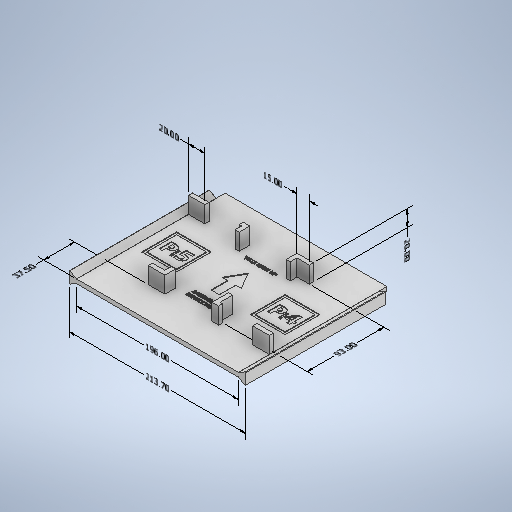
# Autodesk Inventor part: Suelo2
Saved by Autodesk Inventor 2025.1 (Build 291241000, 241)
## iProperties
Created: 2025-11-20
Part Number: Suelo2
Material: Genérico
Document SubType Name: Modeling
Designer: Diego
Density: 1 g/cm^3
Appearance: Valor por defecto
Author: Diego
Autodesk Inventor part; units mm, degrees
(part 1 of 2)
ref_plane "YZ Plane" through (0, 0, 0) normal (1, 0, 0) x (0, 1, 0)
ref_plane "XZ Plane" through (0, 0, 0) normal (0, 1, 0) x (-1, 0, 0)
ref_plane "XY Plane" through (0, 0, 0) normal (0, 0, 1) x (1, 0, 0)
sketch "Boceto1" plane through (0, 0, 0) normal (0, 0, 1) x (1, 0, 0)
  line L0 (-107.4375, 9.96) -> (-116.4375, 15.1562)
  line L1 (-116.4375, 15.1562) -> (-116.4375, -0.2361)
  line L2 (-116.4375, -0.2361) -> (-107.4375, 4.96)
  line L3 (-107.4375, 9.96) -> (-98.4042, 9.96) construction
  line L4 (-107.4375, 4.96) -> (-97.9616, 4.96) construction
  line L5 (-107.4375, 12.46) -> (-107.4375, 9.96) construction
  line L6 (-107.4375, 12.46) -> (-107.4375, 9.96) construction
  line L7 (-107.4375, 2.46) -> (-107.4375, 4.96) construction
  line L8 (88.5625, 12.46) -> (88.5625, 9.96) construction
  line L9 (88.5625, 12.46) -> (88.5625, 9.96) construction
  line L10 (97.5625, -0.2361) -> (88.5625, 4.96)
  line L11 (88.5625, 9.96) -> (97.5625, 15.1562)
  line L12 (97.5625, 15.1562) -> (97.5625, -0.2361)
  line L13 (88.5625, 4.96) -> (88.5625, 4.96) construction
  line L14 (88.5625, 4.96) -> (88.5625, 4.96) construction
  line L15 (88.5625, 4.96) -> (88.5625, 4.96)
  line L16 (88.5625, 7.46) -> (88.5625, 4.96)
  line L17 (88.5625, 4.96) -> (88.5625, 4.96)
  line L18 (88.5625, 9.96) -> (88.5625, 7.46)
  line L19 (-107.4375, 9.96) -> (-107.4375, 4.96)
  point P0 (0, 0)
  point P1 (-116.4375, 7.46)
  point P2 (97.5625, 7.46)
  point P3 (93.0625, 12.5581)
  point P4 (-111.9375, 12.5581)
  dimension "d0" = 60
  constraints: 40 end point, 5 vertical, 3 midpoint, 2 horizontal, 1 collinear, 1 parallel, 5 other
  measures "d0" angle of L0 L1
extrude "Extrusión1" add sketch "Boceto1" against normal blind 170
sketch "Boceto2" plane through (0, 0, 0) normal (0, 0, 1) x (1, 0, 0)
  line L0 (-107.4375, 9.96) -> (-107.4375, 4.96) projected
  line L1 (97.5625, -0.2361) -> (88.5625, 4.96) projected
  line L2 (-107.4375, 9.96) -> (88.5625, 9.96)
  line L3 (88.5625, 9.96) -> (88.5625, 4.96)
  line L4 (88.5625, 4.96) -> (-107.4375, 4.96)
  line L5 (-107.4375, 4.96) -> (-107.4375, 9.96)
  point P0 (0, 0)
  constraints: 8 end point, 2 parallel, 1 horizontal, 1 perpendicular
extrude "Extrusión2" add sketch "Boceto2" against normal blind 180
sketch "Boceto3" plane through (-107.4375, 9.96, 0) normal (0, 1, 0) x (1, 0, 0)
  line L0 (0, 0) -> (196, 0) projected
  line L1 (0, 0) -> (0, 170) projected
  line L2 (0, 180) -> (64.5, 180) construction
  line L3 (64.5, 42.5) -> (0, 42.5) construction
  line L4 (0, 42.5) -> (0, 180) construction
  line L5 (0, 180) -> (196, 180) projected
  line L6 (0, 170) -> (0, 180) projected
  line L7 (196, 180) -> (0, 180) construction
  line L8 (98, 180) -> (98, 0) construction
  line L9 (64.5, 89) -> (0, 89) construction
  line L10 (32.25, 180) -> (32.25, 42.5) construction
  line L11 (64.5, 107) -> (0, 107) construction
  line L12 (64.5, 71) -> (0, 71) construction
  line L13 (64.5, 42.5) -> (64.5, 50.5)
  line L14 (64.5, 50.5) -> (69.5, 50.5)
  line L15 (69.5, 50.5) -> (69.5, 37.5)
  line L16 (69.5, 37.5) -> (49.5, 37.5)
  line L17 (49.5, 37.5) -> (49.5, 42.5)
  line L18 (49.5, 42.5) -> (64.5, 42.5)
  line L19 (64.5, 135.5) -> (64.5, 127.5)
  line L20 (64.5, 127.5) -> (69.5, 127.5)
  line L21 (69.5, 127.5) -> (69.5, 140.5)
  line L22 (69.5, 140.5) -> (64.5, 140.5)
  line L23 (131.5, 42.5) -> (131.5, 57.5)
  line L24 (131.5, 57.5) -> (126.5, 57.5)
  line L25 (126.5, 57.5) -> (126.5, 37.5)
  line L26 (126.5, 37.5) -> (134.5, 37.5)
  line L27 (134.5, 37.5) -> (134.5, 42.5)
  line L28 (134.5, 42.5) -> (131.5, 42.5)
  line L29 (131.5, 127.5) -> (126.5, 127.5)
  line L30 (131.5, 135.5) -> (131.5, 127.5)
  line L31 (146.5, 135.5) -> (131.5, 135.5)
  line L32 (126.5, 135.5) -> (126.5, 140.5)
  line L33 (146.5, 140.5) -> (146.5, 135.5)
  line L34 (126.5, 140.5) -> (146.5, 140.5)
  line L35 (146.5, 140.5) -> (-13.2396, 140.5) construction
  line L36 (0, 140.5) -> (20, 140.5)
  line L37 (20, 140.5) -> (20, 135.5)
  line L38 (20, 135.5) -> (0, 135.5)
  line L39 (0, 135.5) -> (0, 140.5)
  line L40 (64.5, 140.5) -> (61.5, 140.5)
  line L41 (61.5, 140.5) -> (61.5, 135.5)
  line L42 (61.5, 135.5) -> (64.5, 135.5)
  line L43 (64.5, 180) -> (64.5, 140.5) construction
  line L44 (64.5, 135.5) -> (64.5, 42.5) construction
  line L45 (126.5, 135.5) -> (126.5, 127.5)
  line L46 (196, 140.5) -> (176, 140.5) construction
  line L47 (176, 140.5) -> (176, 135.5) construction
  line L48 (176, 135.5) -> (196, 135.5) construction
  line L49 (176, 37.5) -> (176, 42.5)
  line L50 (176, 42.5) -> (196, 42.5)
  line L51 (196, 37.5) -> (176, 37.5)
  line L52 (196, 37.5) -> (196, 42.5)
  point P0 (107.4375, 0)
  point P1 (0, 135.5)
  dimension "d14" = 36
  dimension "d21" = 37.5
  dimension "d22" = 5
  dimension "d23" = 20
  dimension "d24" = 5
  dimension "d25" = 64.5
  dimension "d26" = 13
  dimension "d27" = 46.5
  dimension "d54" = 39.5
  dimension "d60" = 93
  dimension "d76" = 20
  dimension "d77" = 5
  dimension "d81" = 3
  dimension "d82" = 5
  dimension "d83" = 20
  dimension "d84" = 15
  dimension "d85" = 5
  dimension "d89" = 5
  dimension "d90" = 5
  dimension "d93" = 15
  dimension "d94" = 8
  dimension "d95" = 3
  dimension "d97" = 28.5
  dimension "d98" = 5
  dimension "d99" = 5
  constraints: 96 end point, 16 perpendicular, 13 point on line, 11 symmetric about line, 8 horizontal, 6 parallel, 5 midpoint, 5 vertical, 3 collinear, 1 other
  measures "d14" distance between parallel lines of L12 L11
  measures "d21" distance between parallel lines of L0 L16
  measures "d22" distance of L16.end L17.end
  measures "d23" distance of L15.end L16.end
  measures "d24" distance of L13.end L14.end
  measures "d25" distance between parallel lines of L1 L13
  measures "d26" distance of L14.end L15.end
  measures "d27" distance between parallel lines of L18 L9
  measures "d54" distance between parallel lines of L5 L22
  measures "d60" distance between parallel lines of L28 L31
  measures "d76" distance of L37.end L38.end
  measures "d77" distance of L36.end L37.end
  measures "d81" distance of L19.start L41.end
  measures "d82" distance of L40.end L41.end
  measures "d83" distance of L24.end L26.start
  measures "d84" distance of L23.start L24.start
  measures "d85" distance of L24.start L24.end
  measures "d89" distance of L32.start L32.end
  measures "d90" distance of L34.end L31.start
  measures "d93" distance of L31.start L30.start
  measures "d94" distance of L30.start L30.end
  measures "d95" distance of L28.start L23.start
  measures "d97" distance between parallel lines of L8 L25
  measures "d98" distance of L29.start L29.end
  measures "d99" distance of L27.start L28.start
sketch "Boceto4" plane through (-107.4375, 9.96, 0) normal (0, 1, 0) x (1, 0, 0)
  line L0 (12.9564, 122.5347) -> (51.5436, 122.5347) construction
  line L1 (51.5436, 122.5347) -> (51.5436, 55.4653) construction
  line L2 (51.5436, 55.4653) -> (12.9564, 55.4653) construction
  line L3 (12.9564, 55.4653) -> (12.9564, 122.5347) construction
  line L4 (64.5, 107) -> (0, 107) construction
  line L5 (64.5, 89) -> (0, 89) construction
  line L6 (64.5, 71) -> (0, 71) construction
  line L7 (64.5, 180) -> (64.5, 42.5) construction
  line L8 (32.25, 180) -> (32.25, 42.5) construction
  line L9 (98, 180) -> (98, 0) construction
  line L10 (131.5, 107) -> (196, 107) construction
  line L11 (131.5, 89) -> (196, 89) construction
  line L12 (131.5, 71) -> (196, 71) construction
  line L13 (163.75, 180) -> (163.75, 42.5) construction
  line L14 (149.758, 125.112) -> (177.742, 125.112) construction
  line L15 (177.742, 125.112) -> (177.742, 52.888) construction
  line L16 (177.742, 52.888) -> (149.758, 52.888) construction
  line L17 (149.758, 52.888) -> (149.758, 125.112) construction
  line L18 (131.5, 180) -> (131.5, 42.5) construction
  line L19 (14.25, 71) -> (50.25, 71)
  line L20 (50.25, 71) -> (50.25, 107)
  line L21 (50.25, 107) -> (14.25, 107)
  line L22 (14.25, 107) -> (14.25, 71)
  line L23 (14.25, 71) -> (50.25, 107) construction
  line L24 (50.25, 71) -> (14.25, 107) construction
  line L25 (11.25, 68) -> (53.25, 68)
  line L26 (53.25, 68) -> (53.25, 110)
  line L27 (53.25, 110) -> (11.25, 110)
  line L28 (11.25, 110) -> (11.25, 68)
  line L29 (181.75, 71) -> (145.75, 71)
  line L30 (145.75, 71) -> (145.75, 107)
  line L31 (145.75, 107) -> (181.75, 107)
  line L32 (181.75, 107) -> (181.75, 71)
  line L33 (181.75, 71) -> (145.75, 107) construction
  line L34 (145.75, 71) -> (181.75, 107) construction
  line L35 (184.75, 68) -> (142.75, 68)
  line L36 (142.75, 68) -> (142.75, 110)
  line L37 (142.75, 110) -> (184.75, 110)
  line L38 (184.75, 110) -> (184.75, 68)
  line L39 (93, 90) -> (93, 70)
  line L40 (93, 70) -> (103, 70)
  line L41 (103, 70) -> (103, 90)
  line L42 (103, 90) -> (93, 70) construction
  line L43 (93, 90) -> (103, 70) construction
  line L44 (93, 90) -> (86.453, 90)
  line L45 (86.453, 90) -> (98, 110)
  line L46 (98, 110) -> (109.547, 90)
  line L47 (109.547, 90) -> (103, 90)
  line L48 (196, 0) -> (0, 0) projected
  line L49 (74.4962, 55) -> (125.486, 55) construction
  line L50 (82.3818, 77.2089) -> (113.6182, 77.2089) construction
  line L51 (113.6182, 77.2089) -> (113.6182, 32.7911) construction
  line L52 (113.6182, 32.7911) -> (82.3818, 32.7911) construction
  line L53 (82.3818, 32.7911) -> (82.3818, 77.2089) construction
  line L54 (76.287, 55) -> (119.713, 55) construction
  line L55 (98, 110) -> (98, 70) construction
  line L56 (76.287, 125) -> (119.713, 125) construction
  line L57 (78.0417, 136.6375) -> (117.9583, 136.6375) construction
  line L58 (117.9583, 136.6375) -> (117.9583, 113.3625) construction
  line L59 (117.9583, 113.3625) -> (78.0417, 113.3625) construction
  line L60 (78.0417, 113.3625) -> (78.0417, 136.6375) construction
  spline S0 degree 2 poles (29.9202, 91.9295) (29.9202, 90.8841) (29.2516, 88.9878) (28.6317, 88.3558) knots 0 0 0 1 2 2 2
  spline S1 degree 2 poles (28.6317, 88.3558) (28.2549, 87.9546) (27.331, 87.2982) (26.784, 87.0673) knots 0 0 0 1 2 2 2
  spline S2 degree 2 poles (26.784, 87.0673) (26.2249, 86.8363) (24.9242, 86.5689) (24.122, 86.5689) knots 0 0 0 1 2 2 2
  line L61 (24.122, 86.5689) -> (22.1528, 86.5689)
  line L62 (22.1528, 86.5689) -> (22.1528, 81.658)
  line L63 (22.1528, 81.658) -> (18.3845, 81.658)
  line L64 (18.3845, 81.658) -> (18.3845, 96.658)
  line L65 (18.3845, 96.658) -> (24.2071, 96.658)
  spline S3 degree 2 poles (24.2071, 96.658) (25.4955, 96.658) (27.3797, 96.184) (28.1455, 95.6734) knots 0 0 0 1 2 2 2
  spline S4 degree 2 poles (28.1455, 95.6734) (28.9964, 95.1021) (29.9202, 93.2301) (29.9202, 91.9295) knots 0 0 0 1 2 2 2
  spline S5 degree 2 poles (26.0547, 91.8323) (26.0547, 92.4765) (25.4469, 93.3882) (25.0336, 93.5583) knots 0 0 0 1 2 2 2
  spline S6 degree 2 poles (25.0336, 93.5583) (24.4988, 93.7893) (23.5263, 93.8622) (22.6876, 93.8622) knots 0 0 0 1 2 2 2
  line L66 (22.6876, 93.8622) -> (22.1528, 93.8622)
  line L67 (22.1528, 93.8622) -> (22.1528, 89.3647)
  line L68 (22.1528, 89.3647) -> (22.4202, 89.3647)
  spline S7 degree 2 poles (22.4202, 89.3647) (22.9429, 89.3647) (23.891, 89.389) (24.2435, 89.4498) knots 0 0 0 1 2 2 2
  spline S8 degree 2 poles (24.2435, 89.4498) (24.5474, 89.4984) (25.216, 89.7901) (25.3983, 89.9724) knots 0 0 0 1 2 2 2
  spline S9 degree 2 poles (25.3983, 89.9724) (25.7873, 90.3371) (26.0547, 91.1515) (26.0547, 91.8323) knots 0 0 0 1 2 2 2
  line L69 (33.6317, 81.658) -> (31.2816, 81.658)
  line L70 (31.2816, 81.658) -> (31.2816, 89.2026)
  line L71 (31.2816, 89.2026) -> (33.6317, 89.2026)
  line L72 (33.6317, 89.2026) -> (33.6317, 81.658)
  line L73 (33.7046, 90.2804) -> (31.2168, 90.2804)
  line L74 (31.2168, 90.2804) -> (31.2168, 92.1118)
  line L75 (31.2168, 92.1118) -> (33.7046, 92.1118)
  line L76 (33.7046, 92.1118) -> (33.7046, 90.2804)
  spline S10 degree 2 poles (46.7354, 86.7391) (46.7354, 85.56) (45.9331, 83.5665) (45.143, 82.8493) knots 0 0 0 1 2 2 2
  spline S11 degree 2 poles (45.143, 82.8493) (44.3529, 82.1321) (42.1892, 81.342) (40.609, 81.342) knots 0 0 0 1 2 2 2
  spline S12 degree 2 poles (40.609, 81.342) (38.9315, 81.3541) (36.5247, 81.9011) (35.7346, 82.2536) knots 0 0 0 1 2 2 2
  line L77 (35.7346, 82.2536) -> (35.7346, 85.5235)
  line L78 (35.7346, 85.5235) -> (36.075, 85.5235)
  spline S13 degree 2 poles (36.075, 85.5235) (36.3667, 85.3655) (37.0717, 84.9522) (37.643, 84.7334) knots 0 0 0 1 2 2 2
  spline S14 degree 2 poles (37.643, 84.7334) (38.1779, 84.5267) (39.284, 84.2472) (39.9526, 84.2472) knots 0 0 0 1 2 2 2
  spline S15 degree 2 poles (39.9526, 84.2472) (40.5361, 84.2472) (41.8975, 84.5389) (42.3108, 84.9279) knots 0 0 0 1 2 2 2
  spline S16 degree 2 poles (42.3108, 84.9279) (42.6147, 85.2318) (42.955, 85.9733) (42.955, 86.5932) knots 0 0 0 1 2 2 2
  spline S17 degree 2 poles (42.955, 86.5932) (42.955, 87.128) (42.5174, 87.8817) (42.1649, 88.1126) knots 0 0 0 1 2 2 2
  spline S18 degree 2 poles (42.1649, 88.1126) (41.6544, 88.453) (40.1957, 88.6475) (39.673, 88.6475) knots 0 0 0 1 2 2 2
  spline S19 degree 2 poles (39.673, 88.6475) (38.8464, 88.6475) (37.2784, 88.3801) (36.7071, 88.2342) knots 0 0 0 1 2 2 2
  line L79 (36.7071, 88.2342) -> (36.3788, 88.2342)
  line L80 (36.3788, 88.2342) -> (36.3788, 96.658)
  line L81 (36.3788, 96.658) -> (46.3221, 96.658)
  line L82 (46.3221, 96.658) -> (46.3221, 93.8258)
  line L83 (46.3221, 93.8258) -> (39.9404, 93.8258)
  line L84 (39.9404, 93.8258) -> (39.9404, 91.3339)
  spline S20 degree 2 poles (39.9404, 91.3339) (40.2443, 91.3582) (41.0831, 91.3825) (41.314, 91.3825) knots 0 0 0 1 2 2 2
  spline S21 degree 2 poles (41.314, 91.3825) (42.3959, 91.3825) (44.2192, 90.9449) (44.9364, 90.4951) knots 0 0 0 1 2 2 2
  spline S22 degree 2 poles (44.9364, 90.4951) (45.7873, 89.936) (46.7354, 88.0762) (46.7354, 86.7391) knots 0 0 0 1 2 2 2
  spline S23 degree 2 poles (161.4202, 91.7897) (161.4202, 90.7443) (160.7516, 88.8481) (160.1317, 88.216) knots 0 0 0 1 2 2 2
  spline S24 degree 2 poles (160.1317, 88.216) (159.7549, 87.8148) (158.831, 87.1584) (158.284, 86.9275) knots 0 0 0 1 2 2 2
  spline S25 degree 2 poles (158.284, 86.9275) (157.7249, 86.6965) (156.4242, 86.4291) (155.622, 86.4291) knots 0 0 0 1 2 2 2
  line L85 (155.622, 86.4291) -> (153.6528, 86.4291)
  line L86 (153.6528, 86.4291) -> (153.6528, 81.5182)
  line L87 (153.6528, 81.5182) -> (149.8845, 81.5182)
  line L88 (149.8845, 81.5182) -> (149.8845, 96.5182)
  line L89 (149.8845, 96.5182) -> (155.7071, 96.5182)
  spline S26 degree 2 poles (155.7071, 96.5182) (156.9955, 96.5182) (158.8797, 96.0442) (159.6455, 95.5336) knots 0 0 0 1 2 2 2
  spline S27 degree 2 poles (159.6455, 95.5336) (160.4964, 94.9623) (161.4202, 93.0904) (161.4202, 91.7897) knots 0 0 0 1 2 2 2
  spline S28 degree 2 poles (157.5547, 91.6925) (157.5547, 92.3367) (156.9469, 93.2484) (156.5336, 93.4186) knots 0 0 0 1 2 2 2
  spline S29 degree 2 poles (156.5336, 93.4186) (155.9988, 93.6495) (155.0263, 93.7224) (154.1876, 93.7224) knots 0 0 0 1 2 2 2
  line L90 (154.1876, 93.7224) -> (153.6528, 93.7224)
  line L91 (153.6528, 93.7224) -> (153.6528, 89.2249)
  line L92 (153.6528, 89.2249) -> (153.9202, 89.2249)
  spline S30 degree 2 poles (153.9202, 89.2249) (154.4429, 89.2249) (155.391, 89.2492) (155.7435, 89.31) knots 0 0 0 1 2 2 2
  spline S31 degree 2 poles (155.7435, 89.31) (156.0474, 89.3586) (156.716, 89.6503) (156.8983, 89.8327) knots 0 0 0 1 2 2 2
  spline S32 degree 2 poles (156.8983, 89.8327) (157.2873, 90.1973) (157.5547, 91.0118) (157.5547, 91.6925) knots 0 0 0 1 2 2 2
  line L93 (165.1317, 81.5182) -> (162.7816, 81.5182)
  line L94 (162.7816, 81.5182) -> (162.7816, 89.0628)
  line L95 (162.7816, 89.0628) -> (165.1317, 89.0628)
  line L96 (165.1317, 89.0628) -> (165.1317, 81.5182)
  line L97 (165.2046, 90.1406) -> (162.7168, 90.1406)
  line L98 (162.7168, 90.1406) -> (162.7168, 91.972)
  line L99 (162.7168, 91.972) -> (165.2046, 91.972)
  line L100 (165.2046, 91.972) -> (165.2046, 90.1406)
  line L101 (178.7581, 85.019) -> (176.7281, 85.019)
  line L102 (176.7281, 85.019) -> (176.7281, 81.4818)
  line L103 (176.7281, 81.4818) -> (173.0936, 81.4818)
  line L104 (173.0936, 81.4818) -> (173.0936, 85.019)
  line L105 (173.0936, 85.019) -> (166.481, 85.019)
  line L106 (166.481, 85.019) -> (166.481, 87.8148)
  line L107 (166.481, 87.8148) -> (172.972, 96.5182)
  line L108 (172.972, 96.5182) -> (176.7281, 96.5182)
  line L109 (176.7281, 96.5182) -> (176.7281, 87.7176)
  line L110 (176.7281, 87.7176) -> (178.7581, 87.7176)
  line L111 (178.7581, 87.7176) -> (178.7581, 85.019)
  line L112 (173.0936, 87.7176) -> (173.0936, 92.8229)
  line L113 (173.0936, 92.8229) -> (169.2889, 87.7176)
  line L114 (169.2889, 87.7176) -> (173.0936, 87.7176)
  line L115 (83.1118, 56.2994) -> (84.4635, 60.2994)
  line L116 (84.4635, 60.2994) -> (85.5592, 60.2994)
  line L117 (85.5592, 60.2994) -> (86.9109, 56.2994)
  line L118 (86.9109, 56.2994) -> (85.8768, 56.2994)
  line L119 (85.8768, 56.2994) -> (85.6272, 57.1163)
  line L120 (85.6272, 57.1163) -> (84.3695, 57.1163)
  line L121 (84.3695, 57.1163) -> (84.1167, 56.2994)
  line L122 (84.1167, 56.2994) -> (83.1118, 56.2994)
  line L123 (85.4068, 57.8424) -> (84.9984, 59.1649)
  line L124 (84.9984, 59.1649) -> (84.5867, 57.8424)
  line L125 (84.5867, 57.8424) -> (85.4068, 57.8424)
  spline S33 degree 2 poles (88.5446, 56.2281) (88.0843, 56.2281) (87.3906, 56.4064) (87.0924, 56.5361) knots 0 0 0 1 2 2 2
  line L126 (87.0924, 56.5361) -> (87.0924, 57.4891)
  line L127 (87.0924, 57.4891) -> (87.1831, 57.4891)
  spline S34 degree 2 poles (87.1831, 57.4891) (87.4846, 57.233) (88.2075, 56.9575) (88.5478, 56.9575) knots 0 0 0 1 2 2 2
  spline S35 degree 2 poles (88.5478, 56.9575) (88.6353, 56.9575) (88.9173, 56.9964) (89.0016, 57.0352) knots 0 0 0 1 2 2 2
  spline S36 degree 2 poles (89.0016, 57.0352) (89.1053, 57.0806) (89.2512, 57.2459) (89.2512, 57.3788) knots 0 0 0 1 2 2 2
  spline S37 degree 2 poles (89.2512, 57.3788) (89.2512, 57.5312) (89.0146, 57.7192) (88.8525, 57.7613) knots 0 0 0 1 2 2 2
  spline S38 degree 2 poles (88.8525, 57.7613) (88.6483, 57.8164) (88.1848, 57.9105) (87.9806, 57.9818) knots 0 0 0 1 2 2 2
  spline S39 degree 2 poles (87.9806, 57.9818) (87.517, 58.1438) (87.1151, 58.6981) (87.1151, 59.113) knots 0 0 0 1 2 2 2
  spline S40 degree 2 poles (87.1151, 59.113) (87.1151, 59.6738) (88.0648, 60.3707) (88.778, 60.3707) knots 0 0 0 1 2 2 2
  spline S41 degree 2 poles (88.778, 60.3707) (89.1345, 60.3707) (89.8412, 60.2249) (90.1199, 60.1017) knots 0 0 0 1 2 2 2
  line L128 (90.1199, 60.1017) -> (90.1199, 59.1876)
  line L129 (90.1199, 59.1876) -> (90.0324, 59.1876)
  spline S42 degree 2 poles (90.0324, 59.1876) (89.8088, 59.3788) (89.1669, 59.6414) (88.8298, 59.6414) knots 0 0 0 1 2 2 2
  spline S43 degree 2 poles (88.8298, 59.6414) (88.6969, 59.6414) (88.4895, 59.6025) (88.3728, 59.5506) knots 0 0 0 1 2 2 2
  spline S44 degree 2 poles (88.3728, 59.5506) (88.2788, 59.5085) (88.1426, 59.3399) (88.1426, 59.2362) knots 0 0 0 1 2 2 2
  spline S45 degree 2 poles (88.1426, 59.2362) (88.1426, 59.0806) (88.3598, 58.9023) (88.671, 58.831) knots 0 0 0 1 2 2 2
  spline S46 degree 2 poles (88.671, 58.831) (88.872, 58.7857) (89.2447, 58.6981) (89.4587, 58.6236) knots 0 0 0 1 2 2 2
  spline S47 degree 2 poles (89.4587, 58.6236) (89.8736, 58.4712) (90.2788, 57.9656) (90.2788, 57.5506) knots 0 0 0 1 2 2 2
  spline S48 degree 2 poles (90.2788, 57.5506) (90.2788, 56.9542) (89.342, 56.2281) (88.5446, 56.2281) knots 0 0 0 1 2 2 2
  spline S49 degree 2 poles (92.0292, 56.2281) (91.5689, 56.2281) (90.8752, 56.4064) (90.577, 56.5361) knots 0 0 0 1 2 2 2
  line L130 (90.577, 56.5361) -> (90.577, 57.4891)
  line L131 (90.577, 57.4891) -> (90.6677, 57.4891)
  spline S50 degree 2 poles (90.6677, 57.4891) (90.9692, 57.233) (91.6921, 56.9575) (92.0324, 56.9575) knots 0 0 0 1 2 2 2
  spline S51 degree 2 poles (92.0324, 56.9575) (92.1199, 56.9575) (92.4019, 56.9964) (92.4862, 57.0352) knots 0 0 0 1 2 2 2
  spline S52 degree 2 poles (92.4862, 57.0352) (92.59, 57.0806) (92.7358, 57.2459) (92.7358, 57.3788) knots 0 0 0 1 2 2 2
  spline S53 degree 2 poles (92.7358, 57.3788) (92.7358, 57.5312) (92.4992, 57.7192) (92.3371, 57.7613) knots 0 0 0 1 2 2 2
  spline S54 degree 2 poles (92.3371, 57.7613) (92.1329, 57.8164) (91.6694, 57.9105) (91.4652, 57.9818) knots 0 0 0 1 2 2 2
  spline S55 degree 2 poles (91.4652, 57.9818) (91.0016, 58.1438) (90.5997, 58.6981) (90.5997, 59.113) knots 0 0 0 1 2 2 2
  spline S56 degree 2 poles (90.5997, 59.113) (90.5997, 59.6738) (91.5494, 60.3707) (92.2626, 60.3707) knots 0 0 0 1 2 2 2
  spline S57 degree 2 poles (92.2626, 60.3707) (92.6191, 60.3707) (93.3258, 60.2249) (93.6045, 60.1017) knots 0 0 0 1 2 2 2
  line L132 (93.6045, 60.1017) -> (93.6045, 59.1876)
  line L133 (93.6045, 59.1876) -> (93.517, 59.1876)
  spline S58 degree 2 poles (93.517, 59.1876) (93.2934, 59.3788) (92.6515, 59.6414) (92.3144, 59.6414) knots 0 0 0 1 2 2 2
  spline S59 degree 2 poles (92.3144, 59.6414) (92.1815, 59.6414) (91.9741, 59.6025) (91.8574, 59.5506) knots 0 0 0 1 2 2 2
  spline S60 degree 2 poles (91.8574, 59.5506) (91.7634, 59.5085) (91.6272, 59.3399) (91.6272, 59.2362) knots 0 0 0 1 2 2 2
  spline S61 degree 2 poles (91.6272, 59.2362) (91.6272, 59.0806) (91.8444, 58.9023) (92.1556, 58.831) knots 0 0 0 1 2 2 2
  spline S62 degree 2 poles (92.1556, 58.831) (92.3566, 58.7857) (92.7293, 58.6981) (92.9433, 58.6236) knots 0 0 0 1 2 2 2
  spline S63 degree 2 poles (92.9433, 58.6236) (93.3582, 58.4712) (93.7634, 57.9656) (93.7634, 57.5506) knots 0 0 0 1 2 2 2
  spline S64 degree 2 poles (93.7634, 57.5506) (93.7634, 56.9542) (92.8266, 56.2281) (92.0292, 56.2281) knots 0 0 0 1 2 2 2
  line L134 (94.2788, 56.2994) -> (94.2788, 60.2994)
  line L135 (94.2788, 60.2994) -> (96.9822, 60.2994)
  line L136 (96.9822, 60.2994) -> (96.9822, 59.5377)
  line L137 (96.9822, 59.5377) -> (95.2771, 59.5377)
  line L138 (95.2771, 59.5377) -> (95.2771, 58.8343)
  line L139 (95.2771, 58.8343) -> (96.8493, 58.8343)
  line L140 (96.8493, 58.8343) -> (96.8493, 58.0725)
  line L141 (96.8493, 58.0725) -> (95.2771, 58.0725)
  line L142 (95.2771, 58.0725) -> (95.2771, 57.0612)
  line L143 (95.2771, 57.0612) -> (96.9822, 57.0612)
  line L144 (96.9822, 57.0612) -> (96.9822, 56.2994)
  line L145 (96.9822, 56.2994) -> (94.2788, 56.2994)
  line L146 (101.7472, 56.2994) -> (100.7488, 56.2994)
  line L147 (100.7488, 56.2994) -> (100.7488, 58.951)
  line L148 (100.7488, 58.951) -> (100.0227, 57.2395)
  line L149 (100.0227, 57.2395) -> (99.3355, 57.2395)
  line L150 (99.3355, 57.2395) -> (98.6094, 58.951)
  line L151 (98.6094, 58.951) -> (98.6094, 56.2994)
  line L152 (98.6094, 56.2994) -> (97.6629, 56.2994)
  line L153 (97.6629, 56.2994) -> (97.6629, 60.2994)
  line L154 (97.6629, 60.2994) -> (98.8201, 60.2994)
  line L155 (98.8201, 60.2994) -> (99.7083, 58.3254)
  line L156 (99.7083, 58.3254) -> (100.59, 60.2994)
  line L157 (100.59, 60.2994) -> (101.7472, 60.2994)
  line L158 (101.7472, 60.2994) -> (101.7472, 56.2994)
  spline S65 degree 2 poles (105.7731, 57.5247) (105.7731, 57.2265) (105.5462, 56.7759) (105.3582, 56.6268) knots 0 0 0 1 2 2 2
  spline S66 degree 2 poles (105.3582, 56.6268) (105.1313, 56.4485) (104.5932, 56.2994) (104.175, 56.2994) knots 0 0 0 1 2 2 2
  line L159 (104.175, 56.2994) -> (102.577, 56.2994)
  line L160 (102.577, 56.2994) -> (102.577, 60.2994)
  line L161 (102.577, 60.2994) -> (103.987, 60.2994)
  spline S67 degree 2 poles (103.987, 60.2994) (104.4279, 60.2994) (104.8817, 60.2314) (105.0794, 60.1244) knots 0 0 0 1 2 2 2
  spline S68 degree 2 poles (105.0794, 60.1244) (105.2966, 60.0109) (105.5073, 59.622) (105.5073, 59.3691) knots 0 0 0 1 2 2 2
  spline S69 degree 2 poles (105.5073, 59.3691) (105.5073, 59.0774) (105.2156, 58.6203) (104.9562, 58.5134) knots 0 0 0 1 2 2 2
  line L162 (104.9562, 58.5134) -> (104.9562, 58.4939)
  spline S70 degree 2 poles (104.9562, 58.4939) (105.329, 58.4161) (105.7731, 57.9331) (105.7731, 57.5247) knots 0 0 0 1 2 2 2
  spline S71 degree 2 poles (104.7358, 57.5409) (104.7358, 57.7289) (104.5867, 57.9396) (104.4376, 57.9947) knots 0 0 0 1 2 2 2
  spline S72 degree 2 poles (104.4376, 57.9947) (104.3468, 58.0304) (104.0259, 58.0369) (103.7601, 58.0369) knots 0 0 0 1 2 2 2
  line L163 (103.7601, 58.0369) -> (103.5754, 58.0369)
  line L164 (103.5754, 58.0369) -> (103.5754, 57.0288)
  line L165 (103.5754, 57.0288) -> (103.6305, 57.0288)
  spline S73 degree 2 poles (103.6305, 57.0288) (104.0194, 57.0288) (104.3177, 57.0385) (104.4733, 57.1066) knots 0 0 0 1 2 2 2
  spline S74 degree 2 poles (104.4733, 57.1066) (104.6094, 57.1681) (104.7358, 57.3951) (104.7358, 57.5409) knots 0 0 0 1 2 2 2
  spline S75 degree 2 poles (104.4862, 59.1714) (104.4862, 59.2686) (104.3857, 59.4728) (104.282, 59.5182) knots 0 0 0 1 2 2 2
  spline S76 degree 2 poles (104.282, 59.5182) (104.1848, 59.5636) (103.9125, 59.5701) (103.6434, 59.5701) knots 0 0 0 1 2 2 2
  line L166 (103.6434, 59.5701) -> (103.5754, 59.5701)
  line L167 (103.5754, 59.5701) -> (103.5754, 58.7208)
  line L168 (103.5754, 58.7208) -> (103.7018, 58.7208)
  spline S77 degree 2 poles (103.7018, 58.7208) (103.9579, 58.7208) (104.1653, 58.7305) (104.2755, 58.7824) knots 0 0 0 1 2 2 2
  spline S78 degree 2 poles (104.2755, 58.7824) (104.3955, 58.8408) (104.4862, 59.0385) (104.4862, 59.1714) knots 0 0 0 1 2 2 2
  line L169 (109.0178, 56.2994) -> (106.3501, 56.2994)
  line L170 (106.3501, 56.2994) -> (106.3501, 60.2994)
  line L171 (106.3501, 60.2994) -> (107.3549, 60.2994)
  line L172 (107.3549, 60.2994) -> (107.3549, 57.0612)
  line L173 (107.3549, 57.0612) -> (109.0178, 57.0612)
  line L174 (109.0178, 57.0612) -> (109.0178, 56.2994)
  line L175 (112.8233, 60.2994) -> (111.4425, 57.9688)
  line L176 (111.4425, 57.9688) -> (111.4425, 56.2994)
  line L177 (111.4425, 56.2994) -> (110.4376, 56.2994)
  line L178 (110.4376, 56.2994) -> (110.4376, 57.9202)
  line L179 (110.4376, 57.9202) -> (109.034, 60.2994)
  line L180 (109.034, 60.2994) -> (110.1783, 60.2994)
  line L181 (110.1783, 60.2994) -> (110.9595, 58.8732)
  line L182 (110.9595, 58.8732) -> (111.7147, 60.2994)
  line L183 (111.7147, 60.2994) -> (112.8233, 60.2994)
  spline S79 degree 2 poles (85.7958, 51.7103) (85.7958, 51.1495) (85.3063, 50.2678) (84.9335, 50.0312) knots 0 0 0 1 2 2 2
  spline S80 degree 2 poles (84.9335, 50.0312) (84.6224, 49.8302) (83.8898, 49.7135) (83.4781, 49.7135) knots 0 0 0 1 2 2 2
  line L184 (83.4781, 49.7135) -> (82.2269, 49.7135)
  line L185 (82.2269, 49.7135) -> (82.2269, 53.7135)
  line L186 (82.2269, 53.7135) -> (83.4652, 53.7135)
  spline S81 degree 2 poles (83.4652, 53.7135) (83.8865, 53.7135) (84.6224, 53.6066) (84.9465, 53.3991) knots 0 0 0 1 2 2 2
  spline S82 degree 2 poles (84.9465, 53.3991) (85.3387, 53.1463) (85.7958, 52.2905) (85.7958, 51.7103) knots 0 0 0 1 2 2 2
  spline S83 degree 2 poles (84.765, 51.7168) (84.765, 52.1122) (84.4927, 52.6763) (84.2139, 52.8351) knots 0 0 0 1 2 2 2
  spline S84 degree 2 poles (84.2139, 52.8351) (84.0097, 52.9453) (83.5624, 52.968) (83.2512, 52.968) knots 0 0 0 1 2 2 2
  line L187 (83.2512, 52.968) -> (83.2318, 52.968)
  line L188 (83.2318, 52.968) -> (83.2318, 50.4623)
  line L189 (83.2318, 50.4623) -> (83.2512, 50.4623)
  spline S85 degree 2 poles (83.2512, 50.4623) (83.5883, 50.4623) (84.0519, 50.485) (84.2626, 50.6179) knots 0 0 0 1 2 2 2
  spline S86 degree 2 poles (84.2626, 50.6179) (84.5089, 50.7735) (84.765, 51.3213) (84.765, 51.7168) knots 0 0 0 1 2 2 2
  line L190 (88.3825, 49.7135) -> (86.2301, 49.7135)
  line L191 (86.2301, 49.7135) -> (86.2301, 50.4105)
  line L192 (86.2301, 50.4105) -> (86.8039, 50.4105)
  line L193 (86.8039, 50.4105) -> (86.8039, 53.0166)
  line L194 (86.8039, 53.0166) -> (86.2301, 53.0166)
  line L195 (86.2301, 53.0166) -> (86.2301, 53.7135)
  line L196 (86.2301, 53.7135) -> (88.3825, 53.7135)
  line L197 (88.3825, 53.7135) -> (88.3825, 53.0166)
  line L198 (88.3825, 53.0166) -> (87.8088, 53.0166)
  line L199 (87.8088, 53.0166) -> (87.8088, 50.4105)
  line L200 (87.8088, 50.4105) -> (88.3825, 50.4105)
  line L201 (88.3825, 50.4105) -> (88.3825, 49.7135)
  line L202 (92.7455, 49.7135) -> (91.5235, 49.7135)
  line L203 (91.5235, 49.7135) -> (90.4117, 51.1819)
  line L204 (90.4117, 51.1819) -> (90.0486, 51.1819)
  line L205 (90.0486, 51.1819) -> (90.0486, 49.7135)
  line L206 (90.0486, 49.7135) -> (89.0502, 49.7135)
  line L207 (89.0502, 49.7135) -> (89.0502, 53.7135)
  line L208 (89.0502, 53.7135) -> (90.658, 53.7135)
  spline S87 degree 2 poles (90.658, 53.7135) (90.9919, 53.7135) (91.4846, 53.6293) (91.6953, 53.4996) knots 0 0 0 1 2 2 2
  spline S88 degree 2 poles (91.6953, 53.4996) (91.9092, 53.3635) (92.1621, 52.9388) (92.1621, 52.6147) knots 0 0 0 1 2 2 2
  spline S89 degree 2 poles (92.1621, 52.6147) (92.1621, 52.1576) (91.7472, 51.5839) (91.4003, 51.4153) knots 0 0 0 1 2 2 2
  line L209 (91.4003, 51.4153) -> (92.7455, 49.7135)
  spline S90 degree 2 poles (91.1313, 52.4883) (91.1313, 52.6406) (91.0146, 52.8578) (90.8817, 52.9161) knots 0 0 0 1 2 2 2
  spline S91 degree 2 poles (90.8817, 52.9161) (90.7877, 52.955) (90.5575, 52.9777) (90.3857, 52.9777) knots 0 0 0 1 2 2 2
  line L210 (90.3857, 52.9777) -> (90.0486, 52.9777)
  line L211 (90.0486, 52.9777) -> (90.0486, 51.9015)
  line L212 (90.0486, 51.9015) -> (90.3371, 51.9015)
  spline S92 degree 2 poles (90.3371, 51.9015) (90.5446, 51.9015) (90.8395, 51.9534) (90.94, 52.0344) knots 0 0 0 1 2 2 2
  spline S93 degree 2 poles (90.94, 52.0344) (91.0373, 52.1122) (91.1313, 52.3197) (91.1313, 52.4883) knots 0 0 0 1 2 2 2
  line L213 (93.0438, 49.7135) -> (93.0438, 53.7135)
  line L214 (93.0438, 53.7135) -> (95.7472, 53.7135)
  line L215 (95.7472, 53.7135) -> (95.7472, 52.9518)
  line L216 (95.7472, 52.9518) -> (94.0421, 52.9518)
  line L217 (94.0421, 52.9518) -> (94.0421, 52.2484)
  line L218 (94.0421, 52.2484) -> (95.6143, 52.2484)
  line L219 (95.6143, 52.2484) -> (95.6143, 51.4866)
  line L220 (95.6143, 51.4866) -> (94.0421, 51.4866)
  line L221 (94.0421, 51.4866) -> (94.0421, 50.4753)
  line L222 (94.0421, 50.4753) -> (95.7472, 50.4753)
  line L223 (95.7472, 50.4753) -> (95.7472, 49.7135)
  line L224 (95.7472, 49.7135) -> (93.0438, 49.7135)
  spline S94 degree 2 poles (98.1523, 49.6357) (97.2512, 49.6357) (96.1945, 50.7249) (96.1945, 51.7103) knots 0 0 0 1 2 2 2
  spline S95 degree 2 poles (96.1945, 51.7103) (96.1945, 52.6601) (97.2545, 53.7913) (98.1556, 53.7913) knots 0 0 0 1 2 2 2
  spline S96 degree 2 poles (98.1556, 53.7913) (98.3922, 53.7913) (98.7747, 53.7362) (98.9498, 53.6908) knots 0 0 0 1 2 2 2
  spline S97 degree 2 poles (98.9498, 53.6908) (99.0859, 53.6487) (99.4068, 53.5093) (99.5073, 53.4575) knots 0 0 0 1 2 2 2
  line L225 (99.5073, 53.4575) -> (99.5073, 52.5045)
  line L226 (99.5073, 52.5045) -> (99.4068, 52.5045)
  spline S98 degree 2 poles (99.4068, 52.5045) (99.3323, 52.5693) (99.1118, 52.7508) (98.9724, 52.8351) knots 0 0 0 1 2 2 2
  spline S99 degree 2 poles (98.9724, 52.8351) (98.8331, 52.9226) (98.4992, 53.0425) (98.3144, 53.0425) knots 0 0 0 1 2 2 2
  spline S100 degree 2 poles (98.3144, 53.0425) (98.0972, 53.0425) (97.7374, 52.9064) (97.5721, 52.7346) knots 0 0 0 1 2 2 2
  spline S101 degree 2 poles (97.5721, 52.7346) (97.423, 52.5823) (97.2318, 52.0604) (97.2318, 51.7071) knots 0 0 0 1 2 2 2
  spline S102 degree 2 poles (97.2318, 51.7071) (97.2318, 51.3343) (97.4295, 50.8254) (97.5916, 50.6698) knots 0 0 0 1 2 2 2
  spline S103 degree 2 poles (97.5916, 50.6698) (97.7472, 50.5174) (98.1297, 50.3845) (98.3209, 50.3845) knots 0 0 0 1 2 2 2
  spline S104 degree 2 poles (98.3209, 50.3845) (98.5186, 50.3845) (98.8784, 50.5174) (99.0016, 50.5985) knots 0 0 0 1 2 2 2
  spline S105 degree 2 poles (99.0016, 50.5985) (99.1378, 50.6795) (99.342, 50.8513) (99.4165, 50.9194) knots 0 0 0 1 2 2 2
  line L227 (99.4165, 50.9194) -> (99.5073, 50.9194)
  line L228 (99.5073, 50.9194) -> (99.5073, 49.9793)
  spline S106 degree 2 poles (99.5073, 49.9793) (99.3971, 49.9275) (99.1086, 49.7978) (98.953, 49.7524) knots 0 0 0 1 2 2 2
  spline S107 degree 2 poles (98.953, 49.7524) (98.765, 49.6941) (98.4376, 49.6357) (98.1523, 49.6357) knots 0 0 0 1 2 2 2
  line L229 (100.8687, 49.7135) -> (100.8687, 52.9518)
  line L230 (100.8687, 52.9518) -> (99.6856, 52.9518)
  line L231 (99.6856, 52.9518) -> (99.6856, 53.7135)
  line L232 (99.6856, 53.7135) -> (103.0567, 53.7135)
  line L233 (103.0567, 53.7135) -> (103.0567, 52.9518)
  line L234 (103.0567, 52.9518) -> (101.8736, 52.9518)
  line L235 (101.8736, 52.9518) -> (101.8736, 49.7135)
  line L236 (101.8736, 49.7135) -> (100.8687, 49.7135)
  line L237 (105.4587, 49.7135) -> (103.3063, 49.7135)
  line L238 (103.3063, 49.7135) -> (103.3063, 50.4105)
  line L239 (103.3063, 50.4105) -> (103.8801, 50.4105)
  line L240 (103.8801, 50.4105) -> (103.8801, 53.0166)
  line L241 (103.8801, 53.0166) -> (103.3063, 53.0166)
  line L242 (103.3063, 53.0166) -> (103.3063, 53.7135)
  line L243 (103.3063, 53.7135) -> (105.4587, 53.7135)
  line L244 (105.4587, 53.7135) -> (105.4587, 53.0166)
  line L245 (105.4587, 53.0166) -> (104.8849, 53.0166)
  line L246 (104.8849, 53.0166) -> (104.8849, 50.4105)
  line L247 (104.8849, 50.4105) -> (105.4587, 50.4105)
  line L248 (105.4587, 50.4105) -> (105.4587, 49.7135)
  spline S108 degree 2 poles (109.7666, 51.7135) (109.7666, 50.7411) (108.7293, 49.6293) (107.8282, 49.6293) knots 0 0 0 1 2 2 2
  spline S109 degree 2 poles (107.8282, 49.6293) (106.9238, 49.6293) (105.893, 50.7541) (105.893, 51.7135) knots 0 0 0 1 2 2 2
  spline S110 degree 2 poles (105.893, 51.7135) (105.893, 52.6763) (106.9238, 53.7978) (107.8282, 53.7978) knots 0 0 0 1 2 2 2
  spline S111 degree 2 poles (107.8282, 53.7978) (108.7293, 53.7978) (109.7666, 52.6827) (109.7666, 51.7135) knots 0 0 0 1 2 2 2
  spline S112 degree 2 poles (108.7293, 51.7135) (108.7293, 52.0733) (108.5835, 52.5758) (108.457, 52.7346) knots 0 0 0 1 2 2 2
  spline S113 degree 2 poles (108.457, 52.7346) (108.3306, 52.8999) (108.0065, 53.0425) (107.8314, 53.0425) knots 0 0 0 1 2 2 2
  spline S114 degree 2 poles (107.8314, 53.0425) (107.6467, 53.0425) (107.3452, 52.9096) (107.2058, 52.7411) knots 0 0 0 1 2 2 2
  spline S115 degree 2 poles (107.2058, 52.7411) (107.0827, 52.5855) (106.9303, 52.0701) (106.9303, 51.7135) knots 0 0 0 1 2 2 2
  spline S116 degree 2 poles (106.9303, 51.7135) (106.9303, 51.344) (107.0762, 50.8578) (107.2026, 50.6925) knots 0 0 0 1 2 2 2
  spline S117 degree 2 poles (107.2026, 50.6925) (107.329, 50.5272) (107.6564, 50.3845) (107.8314, 50.3845) knots 0 0 0 1 2 2 2
  spline S118 degree 2 poles (107.8314, 50.3845) (108.0097, 50.3845) (108.3404, 50.5369) (108.4603, 50.6989) knots 0 0 0 1 2 2 2
  spline S119 degree 2 poles (108.4603, 50.6989) (108.59, 50.874) (108.7293, 51.3375) (108.7293, 51.7135) knots 0 0 0 1 2 2 2
  line L249 (113.7893, 49.7135) -> (112.8233, 49.7135)
  line L250 (112.8233, 49.7135) -> (111.2804, 52.5012)
  line L251 (111.2804, 52.5012) -> (111.2804, 49.7135)
  line L252 (111.2804, 49.7135) -> (110.363, 49.7135)
  line L253 (110.363, 49.7135) -> (110.363, 53.7135)
  line L254 (110.363, 53.7135) -> (111.5948, 53.7135)
  line L255 (111.5948, 53.7135) -> (112.872, 51.4218)
  line L256 (112.872, 51.4218) -> (112.872, 53.7135)
  line L257 (112.872, 53.7135) -> (113.7893, 53.7135)
  line L258 (113.7893, 53.7135) -> (113.7893, 49.7135)
  line L259 (80.0292, 123.0065) -> (80.0292, 126.2447)
  line L260 (80.0292, 126.2447) -> (78.846, 126.2447)
  line L261 (78.846, 126.2447) -> (78.846, 127.0065)
  line L262 (78.846, 127.0065) -> (82.2172, 127.0065)
  line L263 (82.2172, 127.0065) -> (82.2172, 126.2447)
  line L264 (82.2172, 126.2447) -> (81.034, 126.2447)
  line L265 (81.034, 126.2447) -> (81.034, 123.0065)
  line L266 (81.034, 123.0065) -> (80.0292, 123.0065)
  line L267 (86.0032, 123.0065) -> (84.9984, 123.0065)
  line L268 (84.9984, 123.0065) -> (84.9984, 124.7796)
  line L269 (84.9984, 124.7796) -> (83.6337, 124.7796)
  line L270 (83.6337, 124.7796) -> (83.6337, 123.0065)
  line L271 (83.6337, 123.0065) -> (82.6288, 123.0065)
  line L272 (82.6288, 123.0065) -> (82.6288, 127.0065)
  line L273 (82.6288, 127.0065) -> (83.6337, 127.0065)
  line L274 (83.6337, 127.0065) -> (83.6337, 125.5413)
  line L275 (83.6337, 125.5413) -> (84.9984, 125.5413)
  line L276 (84.9984, 125.5413) -> (84.9984, 127.0065)
  line L277 (84.9984, 127.0065) -> (86.0032, 127.0065)
  line L278 (86.0032, 127.0065) -> (86.0032, 123.0065)
  line L279 (88.8233, 123.0065) -> (86.671, 123.0065)
  line L280 (86.671, 123.0065) -> (86.671, 123.7034)
  line L281 (86.671, 123.7034) -> (87.2447, 123.7034)
  line L282 (87.2447, 123.7034) -> (87.2447, 126.3096)
  line L283 (87.2447, 126.3096) -> (86.671, 126.3096)
  line L284 (86.671, 126.3096) -> (86.671, 127.0065)
  line L285 (86.671, 127.0065) -> (88.8233, 127.0065)
  line L286 (88.8233, 127.0065) -> (88.8233, 126.3096)
  line L287 (88.8233, 126.3096) -> (88.2496, 126.3096)
  line L288 (88.2496, 126.3096) -> (88.2496, 123.7034)
  line L289 (88.2496, 123.7034) -> (88.8233, 123.7034)
  line L290 (88.8233, 123.7034) -> (88.8233, 123.0065)
  spline S120 degree 2 poles (90.7261, 122.9352) (90.2658, 122.9352) (89.5721, 123.1135) (89.2739, 123.2431) knots 0 0 0 1 2 2 2
  line L291 (89.2739, 123.2431) -> (89.2739, 124.1961)
  line L292 (89.2739, 124.1961) -> (89.3647, 124.1961)
  spline S121 degree 2 poles (89.3647, 124.1961) (89.6661, 123.94) (90.389, 123.6645) (90.7293, 123.6645) knots 0 0 0 1 2 2 2
  spline S122 degree 2 poles (90.7293, 123.6645) (90.8169, 123.6645) (91.0989, 123.7034) (91.1831, 123.7423) knots 0 0 0 1 2 2 2
  spline S123 degree 2 poles (91.1831, 123.7423) (91.2869, 123.7877) (91.4327, 123.953) (91.4327, 124.0859) knots 0 0 0 1 2 2 2
  spline S124 degree 2 poles (91.4327, 124.0859) (91.4327, 124.2382) (91.1961, 124.4263) (91.034, 124.4684) knots 0 0 0 1 2 2 2
  spline S125 degree 2 poles (91.034, 124.4684) (90.8298, 124.5235) (90.3663, 124.6175) (90.1621, 124.6888) knots 0 0 0 1 2 2 2
  spline S126 degree 2 poles (90.1621, 124.6888) (89.6985, 124.8509) (89.2966, 125.4052) (89.2966, 125.8201) knots 0 0 0 1 2 2 2
  spline S127 degree 2 poles (89.2966, 125.8201) (89.2966, 126.3809) (90.2464, 127.0778) (90.9595, 127.0778) knots 0 0 0 1 2 2 2
  spline S128 degree 2 poles (90.9595, 127.0778) (91.316, 127.0778) (92.0227, 126.9319) (92.3015, 126.8088) knots 0 0 0 1 2 2 2
  line L293 (92.3015, 126.8088) -> (92.3015, 125.8947)
  line L294 (92.3015, 125.8947) -> (92.2139, 125.8947)
  spline S129 degree 2 poles (92.2139, 125.8947) (91.9903, 126.0859) (91.3485, 126.3485) (91.0113, 126.3485) knots 0 0 0 1 2 2 2
  spline S130 degree 2 poles (91.0113, 126.3485) (90.8784, 126.3485) (90.671, 126.3096) (90.5543, 126.2577) knots 0 0 0 1 2 2 2
  spline S131 degree 2 poles (90.5543, 126.2577) (90.4603, 126.2156) (90.3241, 126.047) (90.3241, 125.9433) knots 0 0 0 1 2 2 2
  spline S132 degree 2 poles (90.3241, 125.9433) (90.3241, 125.7877) (90.5413, 125.6094) (90.8525, 125.5381) knots 0 0 0 1 2 2 2
  spline S133 degree 2 poles (90.8525, 125.5381) (91.0535, 125.4927) (91.4263, 125.4052) (91.6402, 125.3306) knots 0 0 0 1 2 2 2
  spline S134 degree 2 poles (91.6402, 125.3306) (92.0551, 125.1783) (92.4603, 124.6726) (92.4603, 124.2577) knots 0 0 0 1 2 2 2
  spline S135 degree 2 poles (92.4603, 124.2577) (92.4603, 123.6613) (91.5235, 122.9352) (90.7261, 122.9352) knots 0 0 0 1 2 2 2
  spline S136 degree 2 poles (95.8217, 122.9352) (95.3614, 122.9352) (94.6677, 123.1135) (94.3695, 123.2431) knots 0 0 0 1 2 2 2
  line L295 (94.3695, 123.2431) -> (94.3695, 124.1961)
  line L296 (94.3695, 124.1961) -> (94.4603, 124.1961)
  spline S137 degree 2 poles (94.4603, 124.1961) (94.7617, 123.94) (95.4846, 123.6645) (95.825, 123.6645) knots 0 0 0 1 2 2 2
  spline S138 degree 2 poles (95.825, 123.6645) (95.9125, 123.6645) (96.1945, 123.7034) (96.2788, 123.7423) knots 0 0 0 1 2 2 2
  spline S139 degree 2 poles (96.2788, 123.7423) (96.3825, 123.7877) (96.5284, 123.953) (96.5284, 124.0859) knots 0 0 0 1 2 2 2
  spline S140 degree 2 poles (96.5284, 124.0859) (96.5284, 124.2382) (96.2917, 124.4263) (96.1297, 124.4684) knots 0 0 0 1 2 2 2
  spline S141 degree 2 poles (96.1297, 124.4684) (95.9254, 124.5235) (95.4619, 124.6175) (95.2577, 124.6888) knots 0 0 0 1 2 2 2
  spline S142 degree 2 poles (95.2577, 124.6888) (94.7942, 124.8509) (94.3922, 125.4052) (94.3922, 125.8201) knots 0 0 0 1 2 2 2
  spline S143 degree 2 poles (94.3922, 125.8201) (94.3922, 126.3809) (95.342, 127.0778) (96.0551, 127.0778) knots 0 0 0 1 2 2 2
  spline S144 degree 2 poles (96.0551, 127.0778) (96.4117, 127.0778) (97.1183, 126.9319) (97.3971, 126.8088) knots 0 0 0 1 2 2 2
  line L297 (97.3971, 126.8088) -> (97.3971, 125.8947)
  line L298 (97.3971, 125.8947) -> (97.3096, 125.8947)
  spline S145 degree 2 poles (97.3096, 125.8947) (97.0859, 126.0859) (96.4441, 126.3485) (96.107, 126.3485) knots 0 0 0 1 2 2 2
  spline S146 degree 2 poles (96.107, 126.3485) (95.9741, 126.3485) (95.7666, 126.3096) (95.6499, 126.2577) knots 0 0 0 1 2 2 2
  spline S147 degree 2 poles (95.6499, 126.2577) (95.5559, 126.2156) (95.4198, 126.047) (95.4198, 125.9433) knots 0 0 0 1 2 2 2
  spline S148 degree 2 poles (95.4198, 125.9433) (95.4198, 125.7877) (95.637, 125.6094) (95.9481, 125.5381) knots 0 0 0 1 2 2 2
  spline S149 degree 2 poles (95.9481, 125.5381) (96.1491, 125.4927) (96.5219, 125.4052) (96.7358, 125.3306) knots 0 0 0 1 2 2 2
  spline S150 degree 2 poles (96.7358, 125.3306) (97.1507, 125.1783) (97.5559, 124.6726) (97.5559, 124.2577) knots 0 0 0 1 2 2 2
  spline S151 degree 2 poles (97.5559, 124.2577) (97.5559, 123.6613) (96.6191, 122.9352) (95.8217, 122.9352) knots 0 0 0 1 2 2 2
  line L299 (100.0616, 123.0065) -> (97.9092, 123.0065)
  line L300 (97.9092, 123.0065) -> (97.9092, 123.7034)
  line L301 (97.9092, 123.7034) -> (98.483, 123.7034)
  line L302 (98.483, 123.7034) -> (98.483, 126.3096)
  line L303 (98.483, 126.3096) -> (97.9092, 126.3096)
  line L304 (97.9092, 126.3096) -> (97.9092, 127.0065)
  line L305 (97.9092, 127.0065) -> (100.0616, 127.0065)
  line L306 (100.0616, 127.0065) -> (100.0616, 126.3096)
  line L307 (100.0616, 126.3096) -> (99.4878, 126.3096)
  line L308 (99.4878, 126.3096) -> (99.4878, 123.7034)
  line L309 (99.4878, 123.7034) -> (100.0616, 123.7034)
  line L310 (100.0616, 123.7034) -> (100.0616, 123.0065)
  spline S152 degree 2 poles (104.2982, 125.0032) (104.2982, 124.4425) (103.8088, 123.5608) (103.436, 123.3241) knots 0 0 0 1 2 2 2
  spline S153 degree 2 poles (103.436, 123.3241) (103.1248, 123.1232) (102.3922, 123.0065) (101.9806, 123.0065) knots 0 0 0 1 2 2 2
  line L311 (101.9806, 123.0065) -> (100.7293, 123.0065)
  line L312 (100.7293, 123.0065) -> (100.7293, 127.0065)
  line L313 (100.7293, 127.0065) -> (101.9676, 127.0065)
  spline S154 degree 2 poles (101.9676, 127.0065) (102.389, 127.0065) (103.1248, 126.8995) (103.4489, 126.6921) knots 0 0 0 1 2 2 2
  spline S155 degree 2 poles (103.4489, 126.6921) (103.8412, 126.4392) (104.2982, 125.5835) (104.2982, 125.0032) knots 0 0 0 1 2 2 2
  spline S156 degree 2 poles (103.2674, 125.0097) (103.2674, 125.4052) (102.9951, 125.9692) (102.7164, 126.128) knots 0 0 0 1 2 2 2
  spline S157 degree 2 poles (102.7164, 126.128) (102.5122, 126.2382) (102.0648, 126.2609) (101.7536, 126.2609) knots 0 0 0 1 2 2 2
  line L314 (101.7536, 126.2609) -> (101.7342, 126.2609)
  line L315 (101.7342, 126.2609) -> (101.7342, 123.7553)
  line L316 (101.7342, 123.7553) -> (101.7536, 123.7553)
  spline S158 degree 2 poles (101.7536, 123.7553) (102.0908, 123.7553) (102.5543, 123.778) (102.765, 123.9109) knots 0 0 0 1 2 2 2
  spline S159 degree 2 poles (102.765, 123.9109) (103.0113, 124.0665) (103.2674, 124.6143) (103.2674, 125.0097) knots 0 0 0 1 2 2 2
  line L317 (104.8947, 123.0065) -> (104.8947, 127.0065)
  line L318 (104.8947, 127.0065) -> (107.5981, 127.0065)
  line L319 (107.5981, 127.0065) -> (107.5981, 126.2447)
  line L320 (107.5981, 126.2447) -> (105.893, 126.2447)
  line L321 (105.893, 126.2447) -> (105.893, 125.5413)
  line L322 (105.893, 125.5413) -> (107.4652, 125.5413)
  line L323 (107.4652, 125.5413) -> (107.4652, 124.7796)
  line L324 (107.4652, 124.7796) -> (105.893, 124.7796)
  line L325 (105.893, 124.7796) -> (105.893, 123.7682)
  line L326 (105.893, 123.7682) -> (107.5981, 123.7682)
  line L327 (107.5981, 123.7682) -> (107.5981, 123.0065)
  line L328 (107.5981, 123.0065) -> (104.8947, 123.0065)
  spline S160 degree 2 poles (111.5073, 122.9222) (110.7002, 122.9222) (109.8314, 123.7002) (109.8314, 124.4522) knots 0 0 0 1 2 2 2
  line L329 (109.8314, 124.4522) -> (109.8314, 127.0065)
  line L330 (109.8314, 127.0065) -> (110.8363, 127.0065)
  line L331 (110.8363, 127.0065) -> (110.8363, 124.5105)
  spline S161 degree 2 poles (110.8363, 124.5105) (110.8363, 124.0924) (111.1507, 123.684) (111.5073, 123.684) knots 0 0 0 1 2 2 2
  spline S162 degree 2 poles (111.5073, 123.684) (111.8541, 123.684) (112.1783, 124.0762) (112.1783, 124.5105) knots 0 0 0 1 2 2 2
  line L332 (112.1783, 124.5105) -> (112.1783, 127.0065)
  line L333 (112.1783, 127.0065) -> (113.1831, 127.0065)
  line L334 (113.1831, 127.0065) -> (113.1831, 124.4554)
  spline S163 degree 2 poles (113.1831, 124.4554) (113.1831, 123.7164) (112.3371, 122.9222) (111.5073, 122.9222) knots 0 0 0 1 2 2 2
  spline S164 degree 2 poles (117.0308, 125.7455) (117.0308, 125.4668) (116.8525, 124.9611) (116.6872, 124.7925) knots 0 0 0 1 2 2 2
  spline S165 degree 2 poles (116.6872, 124.7925) (116.5867, 124.6856) (116.3404, 124.5105) (116.1945, 124.4489) knots 0 0 0 1 2 2 2
  spline S166 degree 2 poles (116.1945, 124.4489) (116.0454, 124.3874) (115.6985, 124.316) (115.4846, 124.316) knots 0 0 0 1 2 2 2
  line L335 (115.4846, 124.316) -> (114.9595, 124.316)
  line L336 (114.9595, 124.316) -> (114.9595, 123.0065)
  line L337 (114.9595, 123.0065) -> (113.9546, 123.0065)
  line L338 (113.9546, 123.0065) -> (113.9546, 127.0065)
  line L339 (113.9546, 127.0065) -> (115.5073, 127.0065)
  spline S167 degree 2 poles (115.5073, 127.0065) (115.8509, 127.0065) (116.3533, 126.8801) (116.5575, 126.7439) knots 0 0 0 1 2 2 2
  spline S168 degree 2 poles (116.5575, 126.7439) (116.7844, 126.5916) (117.0308, 126.0924) (117.0308, 125.7455) knots 0 0 0 1 2 2 2
  spline S169 degree 2 poles (116, 125.7196) (116, 125.8914) (115.8379, 126.1345) (115.7277, 126.1799) knots 0 0 0 1 2 2 2
  spline S170 degree 2 poles (115.7277, 126.1799) (115.5851, 126.2415) (115.3258, 126.2609) (115.1021, 126.2609) knots 0 0 0 1 2 2 2
  line L340 (115.1021, 126.2609) -> (114.9595, 126.2609)
  line L341 (114.9595, 126.2609) -> (114.9595, 125.0616)
  line L342 (114.9595, 125.0616) -> (115.0308, 125.0616)
  spline S171 degree 2 poles (115.0308, 125.0616) (115.1702, 125.0616) (115.423, 125.0681) (115.517, 125.0843) knots 0 0 0 1 2 2 2
  spline S172 degree 2 poles (115.517, 125.0843) (115.5981, 125.0972) (115.7763, 125.175) (115.825, 125.2237) knots 0 0 0 1 2 2 2
  spline S173 degree 2 poles (115.825, 125.2237) (115.9287, 125.3209) (116, 125.5381) (116, 125.7196) knots 0 0 0 1 2 2 2
  point P0 (107.4375, 0)
  point P1 (32.25, 89)
  point P2 (163.75, 89)
  point P3 (98, 80)
  point P4 (98, 55)
  dimension "d15" = 36
  dimension "d16" = 36
  dimension "d17" = 3
  dimension "d30" = 10
  dimension "d31" = 20
  dimension "d33" = 60
  dimension "d34" = 60
  dimension "d35" = 60
  dimension "d37" = 20
  dimension "d38" = 90
  dimension "d58" = 36
  dimension "d59" = 36
  dimension "d61" = 15
  dimension "d63" = 15
  constraints: 76 end point, 21 symmetric about line, 7 midpoint, 6 equal length, 5 point on line, 4 horizontal, 3 vertical, 2 perpendicular, 19 other
  measures "d15" distance of L21.end L20.end
  measures "d16" distance of L19.end L20.end
  measures "d17" distance between parallel lines of L22 L28
  measures "d30" distance of L39.end L40.end
  measures "d31" distance of L40.end L41.end
  measures "d33" angle of L44 L45
  measures "d34" angle of L47 L46
  measures "d35" angle of L46 L45
  measures "d37" distance from line of L47 L45.end
  measures "d38" distance between parallel lines of L48 L44
  measures "d58" distance of L30.start L30.end
  measures "d59" distance of L30.end L32.start
  measures "d61" distance between parallel lines of L49 L40
  measures "d63" distance between parallel lines of L40 L54
emboss "Repujado1" sketch "Boceto4" operation cut depth 0.8 direction (0, -1, 0)
extrude "Extrusión3" add sketch "Boceto3" along normal blind 20
thicken "Engrosado1" operation cut thickness 0.15 both sides no extend neighbours no toward (-1, 0, 0) faces at (97.5625, 4.8947, -56.6667) (94.5625, 13.4241, -70.8333) (91.5625, 3.228, -113.3333)
thicken "Engrosado2" operation cut thickness 0.15 both sides no extend neighbours no toward (-0.5, -0.8660254, 0) faces at (-113.4375, 13.4241, -101.8333) (-116.4375, 10.0254, -56.6667) (-113.4375, 1.4959, -113.3333)